Autodesk Fusion 360 part; units mm, degrees
note: some values were not read from the file. Chosen so that the rebuilt part matches the saved one: which bodies a step acts on.
(part 2 of 3)
  line L234 (-30.457, -45.4136) -> (-27.043, -43.5255) construction
  line L235 (-27.043, -43.5255) -> (-26.2697, -43.2195) construction
  spline S75 degree 3 poles (-26.2697, -43.2195) (-26.1288, -43.1638) (-26.0775, -43.1652) (-25.9254, -43.2288) knots 0 0 0 0 1 1 1 1
  line L236 (-26.2697, -43.2195) -> (-26.1288, -43.1638) construction
  line L237 (-26.1288, -43.1638) -> (-26.0775, -43.1652) construction
  line L238 (-26.0775, -43.1652) -> (-25.9254, -43.2288) construction
  spline S76 degree 3 poles (-25.9915, -44.0067) (-25.7575, -44.1128) (-24.8189, -44.5936) (-24.3388, -44.8532) knots 0 0 0 0 1 1 1 1
  line L239 (-25.9915, -44.0067) -> (-25.7575, -44.1128) construction
  line L240 (-25.7575, -44.1128) -> (-24.8189, -44.5936) construction
  line L241 (-24.8189, -44.5936) -> (-24.3388, -44.8532) construction
  spline S77 degree 3 poles (-24.3388, -44.8532) (-22.7885, -45.6916) (-21.6552, -46.3596) (-21.7503, -46.379) knots 0 0 0 0 1 1 1 1
  line L242 (-24.3388, -44.8532) -> (-22.7885, -45.6916) construction
  line L243 (-22.7885, -45.6916) -> (-21.6552, -46.3596) construction
  line L244 (-21.6552, -46.3596) -> (-21.7503, -46.379) construction
  spline S78 degree 3 poles (-21.7503, -46.379) (-21.829, -46.395) (-22.3918, -46.1318) (-24.2975, -45.188) knots 0 0 0 0 1 1 1 1
  line L245 (-21.7503, -46.379) -> (-21.829, -46.395) construction
  line L246 (-21.829, -46.395) -> (-22.3918, -46.1318) construction
  line L247 (-22.3918, -46.1318) -> (-24.2975, -45.188) construction
  spline S79 degree 3 poles (-24.2975, -45.188) (-25.1974, -44.7423) (-25.942, -44.3774) (-25.9521, -44.3772) knots 0 0 0 0 1 1 1 1
  line L248 (-24.2975, -45.188) -> (-25.1974, -44.7423) construction
  line L249 (-25.1974, -44.7423) -> (-25.942, -44.3774) construction
  line L250 (-25.942, -44.3774) -> (-25.9521, -44.3772) construction
  spline S80 degree 3 poles (-25.9521, -44.3772) (-25.9622, -44.3769) (-26.5014, -44.6487) (-27.1503, -44.981) knots 0 0 0 0 1 1 1 1
  line L251 (-25.9521, -44.3772) -> (-25.9622, -44.3769) construction
  line L252 (-25.9622, -44.3769) -> (-26.5014, -44.6487) construction
  line L253 (-26.5014, -44.6487) -> (-27.1503, -44.981) construction
  spline S81 degree 3 poles (-27.1503, -44.981) (-28.8926, -45.8734) (-29.5894, -46.2424) (-30.0354, -46.5089) knots 0 0 0 0 1 1 1 1
  line L254 (-27.1503, -44.981) -> (-28.8926, -45.8734) construction
  line L255 (-28.8926, -45.8734) -> (-29.5894, -46.2424) construction
  line L256 (-29.5894, -46.2424) -> (-30.0354, -46.5089) construction
  spline S82 degree 3 poles (-30.0354, -46.5089) (-30.1643, -46.586) (-30.3231, -46.667) (-30.3881, -46.689) knots 0 0 0 0 1 1 1 1
  line L257 (-30.0354, -46.5089) -> (-30.1643, -46.586) construction
  line L258 (-30.1643, -46.586) -> (-30.3231, -46.667) construction
  line L259 (-30.3231, -46.667) -> (-30.3881, -46.689) construction
  spline S83 degree 3 poles (-30.3881, -46.689) (-30.6444, -46.7757) (-30.8249, -46.7116) (-30.7157, -46.5728) knots 0 0 0 0 1 1 1 1
  line L260 (-30.3881, -46.689) -> (-30.6444, -46.7757) construction
  line L261 (-30.6444, -46.7757) -> (-30.8249, -46.7116) construction
  line L262 (-30.8249, -46.7116) -> (-30.7157, -46.5728) construction
  spline S84 degree 3 poles (-30.7157, -46.5728) (-30.5978, -46.4228) (-28.7477, -45.3044) (-27.2723, -44.491) knots 0 0 0 0 1 1 1 1
  line L263 (-30.7157, -46.5728) -> (-30.5978, -46.4228) construction
  line L264 (-30.5978, -46.4228) -> (-28.7477, -45.3044) construction
  line L265 (-28.7477, -45.3044) -> (-27.2723, -44.491) construction
  spline S85 degree 3 poles (-27.2723, -44.491) (-26.8574, -44.2623) (-26.2555, -43.9583) (-26.1898, -43.9443) knots 0 0 0 0 1 1 1 1
  line L266 (-27.2723, -44.491) -> (-26.8574, -44.2623) construction
  line L267 (-26.8574, -44.2623) -> (-26.2555, -43.9583) construction
  line L268 (-26.2555, -43.9583) -> (-26.1898, -43.9443) construction
  spline S86 degree 3 poles (-26.1898, -43.9443) (-26.1622, -43.9384) (-26.0966, -43.959) (-25.9915, -44.0067) knots 0 0 0 0 1 1 1 1
  line L269 (-26.1898, -43.9443) -> (-26.1622, -43.9384) construction
  line L270 (-26.1622, -43.9384) -> (-26.0966, -43.959) construction
  line L271 (-26.0966, -43.959) -> (-25.9915, -44.0067) construction
  spline S87 degree 3 poles (-26.0659, -44.7937) (-25.8421, -44.8752) (-25.0562, -45.2692) (-24.3884, -45.6347) knots 0 0 0 0 1 1 1 1
  line L272 (-26.0659, -44.7937) -> (-25.8421, -44.8752) construction
  line L273 (-25.8421, -44.8752) -> (-25.0562, -45.2692) construction
  line L274 (-25.0562, -45.2692) -> (-24.3884, -45.6347) construction
  spline S88 degree 3 poles (-24.3884, -45.6347) (-23.4262, -46.1613) (-22.272, -46.841) (-22.1077, -46.9777) knots 0 0 0 0 1 1 1 1
  line L275 (-24.3884, -45.6347) -> (-23.4262, -46.1613) construction
  line L276 (-23.4262, -46.1613) -> (-22.272, -46.841) construction
  line L277 (-22.272, -46.841) -> (-22.1077, -46.9777) construction
  line L278 (-22.1077, -46.9777) -> (-22.0664, -47.0121)
  line L279 (-22.0664, -47.0121) -> (-22.1077, -47.0012)
  spline S89 degree 3 poles (-22.1077, -47.0012) (-22.1774, -46.9831) (-22.6584, -46.7746) (-23.0415, -46.5965) knots 0 0 0 0 1 1 1 1
  line L280 (-22.1077, -47.0012) -> (-22.1774, -46.9831) construction
  line L281 (-22.1774, -46.9831) -> (-22.6584, -46.7746) construction
  line L282 (-22.6584, -46.7746) -> (-23.0415, -46.5965) construction
  spline S90 degree 3 poles (-23.0415, -46.5965) (-23.2415, -46.5036) (-23.9837, -46.1421) (-24.691, -45.7932) knots 0 0 0 0 1 1 1 1
  line L283 (-23.0415, -46.5965) -> (-23.2415, -46.5036) construction
  line L284 (-23.2415, -46.5036) -> (-23.9837, -46.1421) construction
  line L285 (-23.9837, -46.1421) -> (-24.691, -45.7932) construction
  spline S91 degree 3 poles (-24.691, -45.7932) (-25.3982, -45.4444) (-25.9848, -45.159) (-25.9944, -45.159) knots 0 0 0 0 1 1 1 1
  line L286 (-24.691, -45.7932) -> (-25.3982, -45.4444) construction
  line L287 (-25.3982, -45.4444) -> (-25.9848, -45.159) construction
  line L288 (-25.9848, -45.159) -> (-25.9944, -45.159) construction
  spline S92 degree 3 poles (-25.9944, -45.159) (-26.0041, -45.159) (-26.5075, -45.4221) (-27.1131, -45.7436) knots 0 0 0 0 1 1 1 1
  line L289 (-25.9944, -45.159) -> (-26.0041, -45.159) construction
  line L290 (-26.0041, -45.159) -> (-26.5075, -45.4221) construction
  line L291 (-26.5075, -45.4221) -> (-27.1131, -45.7436) construction
  spline S93 degree 3 poles (-27.1131, -45.7436) (-29.2269, -46.8659) (-30.1751, -47.357) (-30.2282, -47.357) knots 0 0 0 0 1 1 1 1
  line L292 (-27.1131, -45.7436) -> (-29.2269, -46.8659) construction
  line L293 (-29.2269, -46.8659) -> (-30.1751, -47.357) construction
  line L294 (-30.1751, -47.357) -> (-30.2282, -47.357) construction
  spline S94 degree 3 poles (-30.2282, -47.357) (-30.2637, -47.357) (-30.2915, -47.2851) (-30.2851, -47.2098) knots 0 0 0 0 1 1 1 1
  line L295 (-30.2282, -47.357) -> (-30.2637, -47.357) construction
  line L296 (-30.2637, -47.357) -> (-30.2915, -47.2851) construction
  line L297 (-30.2915, -47.2851) -> (-30.2851, -47.2098) construction
  spline S95 degree 3 poles (-30.2851, -47.2098) (-30.281, -47.1611) (-30.2639, -47.1384) (-30.181, -47.0712) knots 0 0 0 0 1 1 1 1
  line L298 (-30.2851, -47.2098) -> (-30.281, -47.1611) construction
  line L299 (-30.281, -47.1611) -> (-30.2639, -47.1384) construction
  line L300 (-30.2639, -47.1384) -> (-30.181, -47.0712) construction
  spline S96 degree 3 poles (-30.181, -47.0712) (-29.6415, -46.6342) (-26.8805, -45.0293) (-26.2762, -44.8014) knots 0 0 0 0 1 1 1 1
  line L301 (-30.181, -47.0712) -> (-29.6415, -46.6342) construction
  line L302 (-29.6415, -46.6342) -> (-26.8805, -45.0293) construction
  line L303 (-26.8805, -45.0293) -> (-26.2762, -44.8014) construction
  spline S97 degree 3 poles (-26.2762, -44.8014) (-26.154, -44.7553) (-26.1694, -44.7559) (-26.0659, -44.7937) knots 0 0 0 0 1 1 1 1
  line L304 (-26.2762, -44.8014) -> (-26.154, -44.7553) construction
  line L305 (-26.154, -44.7553) -> (-26.1694, -44.7559) construction
  line L306 (-26.1694, -44.7559) -> (-26.0659, -44.7937) construction
  spline S98 degree 3 poles (-25.8841, -45.7204) (-25.6348, -45.7864) (-25.4625, -45.8734) (-24.2727, -46.5342) knots 0 0 0 0 1 1 1 1
  line L307 (-25.8841, -45.7204) -> (-25.6348, -45.7864) construction
  line L308 (-25.6348, -45.7864) -> (-25.4625, -45.8734) construction
  line L309 (-25.4625, -45.8734) -> (-24.2727, -46.5342) construction
  spline S99 degree 3 poles (-24.2727, -46.5342) (-23.1246, -47.1718) (-22.3847, -47.6206) (-22.4583, -47.6347) knots 0 0 0 0 1 1 1 1
  line L310 (-24.2727, -46.5342) -> (-23.1246, -47.1718) construction
  line L311 (-23.1246, -47.1718) -> (-22.3847, -47.6206) construction
  line L312 (-22.3847, -47.6206) -> (-22.4583, -47.6347) construction
  spline S100 degree 3 poles (-22.4583, -47.6347) (-22.4937, -47.6415) (-22.7889, -47.5251) (-23.1407, -47.3656) knots 0 0 0 0 1 1 1 1
  line L313 (-22.4583, -47.6347) -> (-22.4937, -47.6415) construction
  line L314 (-22.4937, -47.6415) -> (-22.7889, -47.5251) construction
  line L315 (-22.7889, -47.5251) -> (-23.1407, -47.3656) construction
  spline S101 degree 3 poles (-23.1407, -47.3656) (-23.4951, -47.2048) (-24.3025, -46.8056) (-25.2404, -46.3275) knots 0 0 0 0 1 1 1 1
  line L316 (-23.1407, -47.3656) -> (-23.4951, -47.2048) construction
  line L317 (-23.4951, -47.2048) -> (-24.3025, -46.8056) construction
  line L318 (-24.3025, -46.8056) -> (-25.2404, -46.3275) construction
  line L319 (-25.2404, -46.3275) -> (-25.9684, -45.9564)
  line L320 (-25.9684, -45.9564) -> (-26.9591, -46.4853)
  spline S102 degree 3 poles (-26.9591, -46.4853) (-28.0366, -47.0606) (-29.1621, -47.6344) (-29.4601, -47.7604) knots 0 0 0 0 1 1 1 1
  line L321 (-26.9591, -46.4853) -> (-28.0366, -47.0606) construction
  line L322 (-28.0366, -47.0606) -> (-29.1621, -47.6344) construction
  line L323 (-29.1621, -47.6344) -> (-29.4601, -47.7604) construction
  spline S103 degree 3 poles (-29.4601, -47.7604) (-29.6667, -47.8478) (-29.7412, -47.8533) (-29.7967, -47.7854) knots 0 0 0 0 1 1 1 1
  line L324 (-29.4601, -47.7604) -> (-29.6667, -47.8478) construction
  line L325 (-29.6667, -47.8478) -> (-29.7412, -47.8533) construction
  line L326 (-29.7412, -47.8533) -> (-29.7967, -47.7854) construction
  spline S104 degree 3 poles (-29.7967, -47.7854) (-29.8338, -47.74) (-29.8332, -47.7011) (-29.7942, -47.625) knots 0 0 0 0 1 1 1 1
  line L327 (-29.7967, -47.7854) -> (-29.8338, -47.74) construction
  line L328 (-29.8338, -47.74) -> (-29.8332, -47.7011) construction
  line L329 (-29.8332, -47.7011) -> (-29.7942, -47.625) construction
  spline S105 degree 3 poles (-29.7942, -47.625) (-29.7453, -47.5297) (-29.7064, -47.5026) (-29.3794, -47.3363) knots 0 0 0 0 1 1 1 1
  line L330 (-29.7942, -47.625) -> (-29.7453, -47.5297) construction
  line L331 (-29.7453, -47.5297) -> (-29.7064, -47.5026) construction
  line L332 (-29.7064, -47.5026) -> (-29.3794, -47.3363) construction
  spline S106 degree 3 poles (-29.3794, -47.3363) (-28.995, -47.1408) (-28.5135, -46.8671) (-27.7433, -46.4059) knots 0 0 0 0 1 1 1 1
  line L333 (-29.3794, -47.3363) -> (-28.995, -47.1408) construction
  line L334 (-28.995, -47.1408) -> (-28.5135, -46.8671) construction
  line L335 (-28.5135, -46.8671) -> (-27.7433, -46.4059) construction
  spline S107 degree 3 poles (-27.7433, -46.4059) (-27.0552, -45.994) (-26.6414, -45.7766) (-26.4448, -45.7237) knots 0 0 0 0 1 1 1 1
  line L336 (-27.7433, -46.4059) -> (-27.0552, -45.994) construction
  line L337 (-27.0552, -45.994) -> (-26.6414, -45.7766) construction
  line L338 (-26.6414, -45.7766) -> (-26.4448, -45.7237) construction
  spline S108 degree 3 poles (-26.4448, -45.7237) (-26.2751, -45.6781) (-26.0486, -45.6767) (-25.8841, -45.7204) knots 0 0 0 0 1 1 1 1
  line L339 (-26.4448, -45.7237) -> (-26.2751, -45.6781) construction
  line L340 (-26.2751, -45.6781) -> (-26.0486, -45.6767) construction
  line L341 (-26.0486, -45.6767) -> (-25.8841, -45.7204) construction
  spline S109 degree 3 poles (-25.8722, -46.4976) (-25.704, -46.5545) (-25.5311, -46.6392) (-25.2843, -46.7853) knots 0 0 0 0 1 1 1 1
  line L342 (-25.8722, -46.4976) -> (-25.704, -46.5545) construction
  line L343 (-25.704, -46.5545) -> (-25.5311, -46.6392) construction
  line L344 (-25.5311, -46.6392) -> (-25.2843, -46.7853) construction
  spline S110 degree 3 poles (-25.2843, -46.7853) (-25.0154, -46.9446) (-24.4604, -47.2593) (-24, -47.5135) knots 0 0 0 0 1 1 1 1
  line L345 (-25.2843, -46.7853) -> (-25.0154, -46.9446) construction
  line L346 (-25.0154, -46.9446) -> (-24.4604, -47.2593) construction
  line L347 (-24.4604, -47.2593) -> (-24, -47.5135) construction
  spline S111 degree 3 poles (-24, -47.5135) (-23.313, -47.8929) (-22.9534, -48.1126) (-22.8762, -48.2001) knots 0 0 0 0 1 1 1 1
  line L348 (-24, -47.5135) -> (-23.313, -47.8929) construction
  line L349 (-23.313, -47.8929) -> (-22.9534, -48.1126) construction
  line L350 (-22.9534, -48.1126) -> (-22.8762, -48.2001) construction
  line L351 (-22.8762, -48.2001) -> (-22.8432, -48.2376)
  line L352 (-22.8432, -48.2376) -> (-22.9087, -48.2256)
  spline S112 degree 3 poles (-22.9087, -48.2256) (-23.1186, -48.1871) (-23.6529, -47.9448) (-24.9223, -47.3123) knots 0 0 0 0 1 1 1 1
  line L353 (-22.9087, -48.2256) -> (-23.1186, -48.1871) construction
  line L354 (-23.1186, -48.1871) -> (-23.6529, -47.9448) construction
  line L355 (-23.6529, -47.9448) -> (-24.9223, -47.3123) construction
  spline S113 degree 3 poles (-24.9223, -47.3123) (-25.475, -47.037) (-25.9351, -46.8117) (-25.9447, -46.8117) knots 0 0 0 0 1 1 1 1
  line L356 (-24.9223, -47.3123) -> (-25.475, -47.037) construction
  line L357 (-25.475, -47.037) -> (-25.9351, -46.8117) construction
  line L358 (-25.9351, -46.8117) -> (-25.9447, -46.8117) construction
  spline S114 degree 3 poles (-25.9447, -46.8117) (-25.9544, -46.8117) (-26.2794, -46.9746) (-26.6669, -47.1737) knots 0 0 0 0 1 1 1 1
  line L359 (-25.9447, -46.8117) -> (-25.9544, -46.8117) construction
  line L360 (-25.9544, -46.8117) -> (-26.2794, -46.9746) construction
  line L361 (-26.2794, -46.9746) -> (-26.6669, -47.1737) construction
  spline S115 degree 3 poles (-26.6669, -47.1737) (-28.0497, -47.8842) (-28.5938, -48.1478) (-29.0112, -48.3091) knots 0 0 0 0 1 1 1 1
  line L362 (-26.6669, -47.1737) -> (-28.0497, -47.8842) construction
  line L363 (-28.0497, -47.8842) -> (-28.5938, -48.1478) construction
  line L364 (-28.5938, -48.1478) -> (-29.0112, -48.3091) construction
  spline S116 degree 3 poles (-29.0112, -48.3091) (-29.1142, -48.3489) (-29.2276, -48.3861) (-29.2633, -48.3918) knots 0 0 0 0 1 1 1 1
  line L365 (-29.0112, -48.3091) -> (-29.1142, -48.3489) construction
  line L366 (-29.1142, -48.3489) -> (-29.2276, -48.3861) construction
  line L367 (-29.2276, -48.3861) -> (-29.2633, -48.3918) construction
  spline S117 degree 3 poles (-29.2633, -48.3918) (-29.3229, -48.4013) (-29.3291, -48.3987) (-29.3388, -48.3601) knots 0 0 0 0 1 1 1 1
  line L368 (-29.2633, -48.3918) -> (-29.3229, -48.4013) construction
  line L369 (-29.3229, -48.4013) -> (-29.3291, -48.3987) construction
  line L370 (-29.3291, -48.3987) -> (-29.3388, -48.3601) construction
  spline S118 degree 3 poles (-29.3388, -48.3601) (-29.3638, -48.2604) (-29.29, -48.1741) (-29.033, -48.0024) knots 0 0 0 0 1 1 1 1
  line L371 (-29.3388, -48.3601) -> (-29.3638, -48.2604) construction
  line L372 (-29.3638, -48.2604) -> (-29.29, -48.1741) construction
  line L373 (-29.29, -48.1741) -> (-29.033, -48.0024) construction
  spline S119 degree 3 poles (-29.033, -48.0024) (-28.4019, -47.5806) (-26.7702, -46.6937) (-26.2531, -46.4912) knots 0 0 0 0 1 1 1 1
  line L374 (-29.033, -48.0024) -> (-28.4019, -47.5806) construction
  line L375 (-28.4019, -47.5806) -> (-26.7702, -46.6937) construction
  line L376 (-26.7702, -46.6937) -> (-26.2531, -46.4912) construction
  spline S120 degree 3 poles (-26.2531, -46.4912) (-26.1127, -46.4363) (-26.05, -46.4373) (-25.8722, -46.4976) knots 0 0 0 0 1 1 1 1
  line L377 (-26.2531, -46.4912) -> (-26.1127, -46.4363) construction
  line L378 (-26.1127, -46.4363) -> (-26.05, -46.4373) construction
  line L379 (-26.05, -46.4373) -> (-25.8722, -46.4976) construction
  spline S121 degree 3 poles (-26.0328, -47.2597) (-25.9016, -47.3132) (-25.2551, -47.6361) (-24.8759, -47.8375) knots 0 0 0 0 1 1 1 1
  line L380 (-26.0328, -47.2597) -> (-25.9016, -47.3132) construction
  line L381 (-25.9016, -47.3132) -> (-25.2551, -47.6361) construction
  line L382 (-25.2551, -47.6361) -> (-24.8759, -47.8375) construction
  spline S122 degree 3 poles (-24.8759, -47.8375) (-24.0296, -48.287) (-23.2843, -48.7426) (-23.3689, -48.7589) knots 0 0 0 0 1 1 1 1
  line L383 (-24.8759, -47.8375) -> (-24.0296, -48.287) construction
  line L384 (-24.0296, -48.287) -> (-23.2843, -48.7426) construction
  line L385 (-23.2843, -48.7426) -> (-23.3689, -48.7589) construction
  spline S123 degree 3 poles (-23.3689, -48.7589) (-23.4678, -48.7779) (-24.1054, -48.5) (-25.271, -47.9296) knots 0 0 0 0 1 1 1 1
  line L386 (-23.3689, -48.7589) -> (-23.4678, -48.7779) construction
  line L387 (-23.4678, -48.7779) -> (-24.1054, -48.5) construction
  line L388 (-24.1054, -48.5) -> (-25.271, -47.9296) construction
  spline S124 degree 3 poles (-25.271, -47.9296) (-25.7194, -47.7101) (-25.9049, -47.627) (-25.9238, -47.6371) knots 0 0 0 0 1 1 1 1
  line L389 (-25.271, -47.9296) -> (-25.7194, -47.7101) construction
  line L390 (-25.7194, -47.7101) -> (-25.9049, -47.627) construction
  line L391 (-25.9049, -47.627) -> (-25.9238, -47.6371) construction
  spline S125 degree 3 poles (-25.9238, -47.6371) (-25.9986, -47.6768) (-27.5715, -48.4353) (-27.7846, -48.5344) knots 0 0 0 0 1 1 1 1
  line L392 (-25.9238, -47.6371) -> (-25.9986, -47.6768) construction
  line L393 (-25.9986, -47.6768) -> (-27.5715, -48.4353) construction
  line L394 (-27.5715, -48.4353) -> (-27.7846, -48.5344) construction
  spline S126 degree 3 poles (-27.7846, -48.5344) (-28.514, -48.8736) (-28.7769, -48.9621) (-28.8571, -48.8955) knots 0 0 0 0 1 1 1 1
  line L395 (-27.7846, -48.5344) -> (-28.514, -48.8736) construction
  line L396 (-28.514, -48.8736) -> (-28.7769, -48.9621) construction
  line L397 (-28.7769, -48.9621) -> (-28.8571, -48.8955) construction
  spline S127 degree 3 poles (-28.8571, -48.8955) (-28.9273, -48.8372) (-28.8768, -48.7847) (-28.5319, -48.5575) knots 0 0 0 0 1 1 1 1
  line L398 (-28.8571, -48.8955) -> (-28.9273, -48.8372) construction
  line L399 (-28.9273, -48.8372) -> (-28.8768, -48.7847) construction
  line L400 (-28.8768, -48.7847) -> (-28.5319, -48.5575) construction
  spline S128 degree 3 poles (-28.5319, -48.5575) (-27.7923, -48.0703) (-26.3775, -47.2824) (-26.1567, -47.2348) knots 0 0 0 0 1 1 1 1
  line L401 (-28.5319, -48.5575) -> (-27.7923, -48.0703) construction
  line L402 (-27.7923, -48.0703) -> (-26.3775, -47.2824) construction
  line L403 (-26.3775, -47.2824) -> (-26.1567, -47.2348) construction
  spline S129 degree 3 poles (-26.1567, -47.2348) (-26.1335, -47.2299) (-26.0794, -47.2407) (-26.0328, -47.2597) knots 0 0 0 0 1 1 1 1
  line L404 (-26.1567, -47.2348) -> (-26.1335, -47.2299) construction
  line L405 (-26.1335, -47.2299) -> (-26.0794, -47.2407) construction
  line L406 (-26.0794, -47.2407) -> (-26.0328, -47.2597) construction
  spline S130 degree 3 poles (-25.9006, -48.1072) (-25.2283, -48.4297) (-23.942, -49.1704) (-23.8197, -49.3056) knots 0 0 0 0 1 1 1 1
  line L407 (-25.9006, -48.1072) -> (-25.2283, -48.4297) construction
  line L408 (-25.2283, -48.4297) -> (-23.942, -49.1704) construction
  line L409 (-23.942, -49.1704) -> (-23.8197, -49.3056) construction
  spline S131 degree 3 poles (-23.8197, -49.3056) (-23.7888, -49.3397) (-23.7889, -49.3402) (-23.8227, -49.3402) knots 0 0 0 0 1 1 1 1
  line L410 (-23.8197, -49.3056) -> (-23.7888, -49.3397) construction
  line L411 (-23.7888, -49.3397) -> (-23.7889, -49.3402) construction
  line L412 (-23.7889, -49.3402) -> (-23.8227, -49.3402) construction
  spline S132 degree 3 poles (-23.8227, -49.3402) (-23.9179, -49.3402) (-24.4007, -49.144) (-25.2495, -48.7602) knots 0 0 0 0 1 1 1 1
  line L413 (-23.8227, -49.3402) -> (-23.9179, -49.3402) construction
  line L414 (-23.9179, -49.3402) -> (-24.4007, -49.144) construction
  line L415 (-24.4007, -49.144) -> (-25.2495, -48.7602) construction
  spline S133 degree 3 poles (-25.2495, -48.7602) (-25.6094, -48.5975) (-25.913, -48.4643) (-25.924, -48.4643) knots 0 0 0 0 1 1 1 1
  line L416 (-25.2495, -48.7602) -> (-25.6094, -48.5975) construction
  line L417 (-25.6094, -48.5975) -> (-25.913, -48.4643) construction
  line L418 (-25.913, -48.4643) -> (-25.924, -48.4643) construction
  spline S134 degree 3 poles (-25.924, -48.4643) (-25.935, -48.4643) (-26.2244, -48.5991) (-26.5669, -48.7639) knots 0 0 0 0 1 1 1 1
  line L419 (-25.924, -48.4643) -> (-25.935, -48.4643) construction
  line L420 (-25.935, -48.4643) -> (-26.2244, -48.5991) construction
  line L421 (-26.2244, -48.5991) -> (-26.5669, -48.7639) construction
  spline S135 degree 3 poles (-26.5669, -48.7639) (-27.3036, -49.1182) (-27.5407, -49.2246) (-27.849, -49.3392) knots 0 0 0 0 1 1 1 1
  line L422 (-26.5669, -48.7639) -> (-27.3036, -49.1182) construction
  line L423 (-27.3036, -49.1182) -> (-27.5407, -49.2246) construction
  line L424 (-27.5407, -49.2246) -> (-27.849, -49.3392) construction
  spline S136 degree 3 poles (-27.849, -49.3392) (-28.0734, -49.4226) (-28.3094, -49.4887) (-28.3838, -49.4889) knots 0 0 0 0 1 1 1 1
  line L425 (-27.849, -49.3392) -> (-28.0734, -49.4226) construction
  line L426 (-28.0734, -49.4226) -> (-28.3094, -49.4887) construction
  line L427 (-28.3094, -49.4887) -> (-28.3838, -49.4889) construction
  spline S137 degree 3 poles (-28.3838, -49.4889) (-28.5219, -49.4894) (-28.2585, -49.2609) (-27.669, -48.8691) knots 0 0 0 0 1 1 1 1
  line L428 (-28.3838, -49.4889) -> (-28.5219, -49.4894) construction
  line L429 (-28.5219, -49.4894) -> (-28.2585, -49.2609) construction
  line L430 (-28.2585, -49.2609) -> (-27.669, -48.8691) construction
  spline S138 degree 3 poles (-27.669, -48.8691) (-26.9446, -48.3877) (-26.2659, -48.0154) (-26.1193, -48.0191) knots 0 0 0 0 1 1 1 1
  line L431 (-27.669, -48.8691) -> (-26.9446, -48.3877) construction
  line L432 (-26.9446, -48.3877) -> (-26.2659, -48.0154) construction
  line L433 (-26.2659, -48.0154) -> (-26.1193, -48.0191) construction
  spline S139 degree 3 poles (-26.1193, -48.0191) (-26.099, -48.0195) (-26.0006, -48.0592) (-25.9006, -48.1072) knots 0 0 0 0 1 1 1 1
  line L434 (-26.1193, -48.0191) -> (-26.099, -48.0195) construction
  line L435 (-26.099, -48.0195) -> (-26.0006, -48.0592) construction
  line L436 (-26.0006, -48.0592) -> (-25.9006, -48.1072) construction
  spline S140 degree 3 poles (-25.9254, -48.9692) (-25.8145, -48.9977) (-24.4971, -49.6532) (-24.3171, -49.7694) knots 0 0 0 0 1 1 1 1
  line L437 (-25.9254, -48.9692) -> (-25.8145, -48.9977) construction
  line L438 (-25.8145, -48.9977) -> (-24.4971, -49.6532) construction
  line L439 (-24.4971, -49.6532) -> (-24.3171, -49.7694) construction
  spline S141 degree 3 poles (-24.3171, -49.7694) (-24.202, -49.8437) (-24.1885, -49.8578) (-24.1931, -49.8982) knots 0 0 0 0 1 1 1 1
  line L440 (-24.3171, -49.7694) -> (-24.202, -49.8437) construction
  line L441 (-24.202, -49.8437) -> (-24.1885, -49.8578) construction
  line L442 (-24.1885, -49.8578) -> (-24.1931, -49.8982) construction
  spline S142 degree 3 poles (-24.1931, -49.8982) (-24.2002, -49.959) (-24.2445, -49.9635) (-24.3936, -49.9184) knots 0 0 0 0 1 1 1 1
  line L443 (-24.1931, -49.8982) -> (-24.2002, -49.959) construction
  line L444 (-24.2002, -49.959) -> (-24.2445, -49.9635) construction
  line L445 (-24.2445, -49.9635) -> (-24.3936, -49.9184) construction
  spline S143 degree 3 poles (-24.3936, -49.9184) (-24.5983, -49.8565) (-24.875, -49.7409) (-25.4105, -49.4935) knots 0 0 0 0 1 1 1 1
  line L446 (-24.3936, -49.9184) -> (-24.5983, -49.8565) construction
  line L447 (-24.5983, -49.8565) -> (-24.875, -49.7409) construction
  line L448 (-24.875, -49.7409) -> (-25.4105, -49.4935) construction
  line L449 (-25.4105, -49.4935) -> (-25.9286, -49.2542)
  line L450 (-25.9286, -49.2542) -> (-26.5095, -49.5354)
  spline S144 degree 3 poles (-26.5095, -49.5354) (-27.3555, -49.9449) (-27.6003, -50.0371) (-27.8507, -50.0406) knots 0 0 0 0 1 1 1 1
  line L451 (-26.5095, -49.5354) -> (-27.3555, -49.9449) construction
  line L452 (-27.3555, -49.9449) -> (-27.6003, -50.0371) construction
  line L453 (-27.6003, -50.0371) -> (-27.8507, -50.0406) construction
  spline S145 degree 3 poles (-27.8507, -50.0406) (-27.9926, -50.0425) (-27.9997, -50.0409) (-28.0047, -50.0059) knots 0 0 0 0 1 1 1 1
  line L454 (-27.8507, -50.0406) -> (-27.9926, -50.0425) construction
  line L455 (-27.9926, -50.0425) -> (-27.9997, -50.0409) construction
  line L456 (-27.9997, -50.0409) -> (-28.0047, -50.0059) construction
  spline S146 degree 3 poles (-28.0047, -50.0059) (-28.012, -49.9538) (-27.8877, -49.8263) (-27.7128, -49.7065) knots 0 0 0 0 1 1 1 1
  line L457 (-28.0047, -50.0059) -> (-28.012, -49.9538) construction
  line L458 (-28.012, -49.9538) -> (-27.8877, -49.8263) construction
  line L459 (-27.8877, -49.8263) -> (-27.7128, -49.7065) construction
  spline S147 degree 3 poles (-27.7128, -49.7065) (-27.5513, -49.596) (-26.8845, -49.2091) (-26.6652, -49.0988) knots 0 0 0 0 1 1 1 1
  line L460 (-27.7128, -49.7065) -> (-27.5513, -49.596) construction
  line L461 (-27.5513, -49.596) -> (-26.8845, -49.2091) construction
  line L462 (-26.8845, -49.2091) -> (-26.6652, -49.0988) construction
  spline S148 degree 3 poles (-26.6652, -49.0988) (-26.3641, -48.9473) (-26.1537, -48.9104) (-25.9254, -48.9692) knots 0 0 0 0 1 1 1 1
  line L463 (-26.6652, -49.0988) -> (-26.3641, -48.9473) construction
  line L464 (-26.3641, -48.9473) -> (-26.1537, -48.9104) construction
  line L465 (-26.1537, -48.9104) -> (-25.9254, -48.9692) construction
  spline S149 degree 3 poles (-25.8427, -49.7941) (-25.6795, -49.8407) (-25.3299, -50.0067) (-25.0638, -50.164) knots 0 0 0 0 1 1 1 1
  line L466 (-25.8427, -49.7941) -> (-25.6795, -49.8407) construction
  line L467 (-25.6795, -49.8407) -> (-25.3299, -50.0067) construction
  line L468 (-25.3299, -50.0067) -> (-25.0638, -50.164) construction
  spline S150 degree 3 poles (-25.0638, -50.164) (-24.796, -50.3224) (-24.6972, -50.4481) (-24.8306, -50.461) knots 0 0 0 0 1 1 1 1
  line L469 (-25.0638, -50.164) -> (-24.796, -50.3224) construction
  line L470 (-24.796, -50.3224) -> (-24.6972, -50.4481) construction
  line L471 (-24.6972, -50.4481) -> (-24.8306, -50.461) construction
  spline S151 degree 3 poles (-24.8306, -50.461) (-24.9117, -50.4688) (-25.1331, -50.4077) (-25.3984, -50.3043) knots 0 0 0 0 1 1 1 1
  line L472 (-24.8306, -50.461) -> (-24.9117, -50.4688) construction
  line L473 (-24.9117, -50.4688) -> (-25.1331, -50.4077) construction
  line L474 (-25.1331, -50.4077) -> (-25.3984, -50.3043) construction
  spline S152 degree 3 poles (-25.3984, -50.3043) (-25.699, -50.1871) (-25.7745, -50.167) (-25.9147, -50.1668) knots 0 0 0 0 1 1 1 1
  line L475 (-25.3984, -50.3043) -> (-25.699, -50.1871) construction
  line L476 (-25.699, -50.1871) -> (-25.7745, -50.167) construction
  line L477 (-25.7745, -50.167) -> (-25.9147, -50.1668) construction
  spline S153 degree 3 poles (-25.9147, -50.1668) (-26.0765, -50.1665) (-26.1933, -50.2019) (-26.5139, -50.3483) knots 0 0 0 0 1 1 1 1
  line L478 (-25.9147, -50.1668) -> (-26.0765, -50.1665) construction
  line L479 (-26.0765, -50.1665) -> (-26.1933, -50.2019) construction
  line L480 (-26.1933, -50.2019) -> (-26.5139, -50.3483) construction
  spline S154 degree 3 poles (-26.5139, -50.3483) (-26.9633, -50.5536) (-27.2052, -50.6374) (-27.4045, -50.6567) knots 0 0 0 0 1 1 1 1
  line L481 (-26.5139, -50.3483) -> (-26.9633, -50.5536) construction
  line L482 (-26.9633, -50.5536) -> (-27.2052, -50.6374) construction
  line L483 (-27.2052, -50.6374) -> (-27.4045, -50.6567) construction
  spline S155 degree 3 poles (-27.4045, -50.6567) (-27.4871, -50.6646) (-27.5102, -50.6609) (-27.5429, -50.6344) knots 0 0 0 0 1 1 1 1
  line L484 (-27.4045, -50.6567) -> (-27.4871, -50.6646) construction
  line L485 (-27.4871, -50.6646) -> (-27.5102, -50.6609) construction
  line L486 (-27.5102, -50.6609) -> (-27.5429, -50.6344) construction
  spline S156 degree 3 poles (-27.5429, -50.6344) (-27.5806, -50.6038) (-27.5811, -50.6005) (-27.556, -50.552) knots 0 0 0 0 1 1 1 1
  line L487 (-27.5429, -50.6344) -> (-27.5806, -50.6038) construction
  line L488 (-27.5806, -50.6038) -> (-27.5811, -50.6005) construction
  line L489 (-27.5811, -50.6005) -> (-27.556, -50.552) construction
  spline S157 degree 3 poles (-27.556, -50.552) (-27.5229, -50.4881) (-27.3926, -50.3704) (-27.2502, -50.276) knots 0 0 0 0 1 1 1 1
  line L490 (-27.556, -50.552) -> (-27.5229, -50.4881) construction
  line L491 (-27.5229, -50.4881) -> (-27.3926, -50.3704) construction
  line L492 (-27.3926, -50.3704) -> (-27.2502, -50.276) construction
  spline S158 degree 3 poles (-27.2502, -50.276) (-26.9831, -50.0988) (-26.4712, -49.8463) (-26.2771, -49.796) knots 0 0 0 0 1 1 1 1
  line L493 (-27.2502, -50.276) -> (-26.9831, -50.0988) construction
  line L494 (-26.9831, -50.0988) -> (-26.4712, -49.8463) construction
  line L495 (-26.4712, -49.8463) -> (-26.2771, -49.796) construction
  spline S159 degree 3 poles (-26.2771, -49.796) (-26.1585, -49.7652) (-25.9473, -49.7643) (-25.8427, -49.7941) knots 0 0 0 0 1 1 1 1
  line L496 (-26.2771, -49.796) -> (-26.1585, -49.7652) construction
  line L497 (-26.1585, -49.7652) -> (-25.9473, -49.7643) construction
  line L498 (-25.9473, -49.7643) -> (-25.8427, -49.7941) construction
  spline S160 degree 3 poles (-26.0163, -50.55) (-25.7916, -50.6279) (-25.2799, -50.9167) (-25.2232, -50.9977) knots 0 0 0 0 1 1 1 1
  line L499 (-26.0163, -50.55) -> (-25.7916, -50.6279) construction
  line L500 (-25.7916, -50.6279) -> (-25.2799, -50.9167) construction
  line L501 (-25.2799, -50.9167) -> (-25.2232, -50.9977) construction
  spline S161 degree 3 poles (-25.2232, -50.9977) (-25.143, -51.1121) (-25.2749, -51.1127) (-25.6038, -50.9992) knots 0 0 0 0 1 1 1 1
  line L502 (-25.2232, -50.9977) -> (-25.143, -51.1121) construction
  line L503 (-25.143, -51.1121) -> (-25.2749, -51.1127) construction
  line L504 (-25.2749, -51.1127) -> (-25.6038, -50.9992) construction
  spline S162 degree 3 poles (-25.6038, -50.9992) (-25.713, -50.9615) (-25.7633, -50.9538) (-25.9006, -50.9538) knots 0 0 0 0 1 1 1 1
  line L505 (-25.6038, -50.9992) -> (-25.713, -50.9615) construction
  line L506 (-25.713, -50.9615) -> (-25.7633, -50.9538) construction
  line L507 (-25.7633, -50.9538) -> (-25.9006, -50.9538) construction
  spline S163 degree 3 poles (-25.9006, -50.9538) (-26.0871, -50.9538) (-26.2188, -50.9903) (-26.4505, -51.1065) knots 0 0 0 0 1 1 1 1
  line L508 (-25.9006, -50.9538) -> (-26.0871, -50.9538) construction
  line L509 (-26.0871, -50.9538) -> (-26.2188, -50.9903) construction
  line L510 (-26.2188, -50.9903) -> (-26.4505, -51.1065) construction
  spline S164 degree 3 poles (-26.4505, -51.1065) (-26.7236, -51.2434) (-26.9716, -51.3032) (-27.0801, -51.2582) knots 0 0 0 0 1 1 1 1
  line L511 (-26.4505, -51.1065) -> (-26.7236, -51.2434) construction
  line L512 (-26.7236, -51.2434) -> (-26.9716, -51.3032) construction
  line L513 (-26.9716, -51.3032) -> (-27.0801, -51.2582) construction
  spline S165 degree 3 poles (-27.0801, -51.2582) (-27.1388, -51.2339) (-27.1754, -51.1592) (-27.151, -51.1135) knots 0 0 0 0 1 1 1 1
  line L514 (-27.0801, -51.2582) -> (-27.1388, -51.2339) construction
  line L515 (-27.1388, -51.2339) -> (-27.1754, -51.1592) construction
  line L516 (-27.1754, -51.1592) -> (-27.151, -51.1135) construction
  spline S166 degree 3 poles (-27.151, -51.1135) (-27.0975, -51.0135) (-26.8146, -50.8094) (-26.5369, -50.6703) knots 0 0 0 0 1 1 1 1
  line L517 (-27.151, -51.1135) -> (-27.0975, -51.0135) construction
  line L518 (-27.0975, -51.0135) -> (-26.8146, -50.8094) construction
  line L519 (-26.8146, -50.8094) -> (-26.5369, -50.6703) construction
  spline S167 degree 3 poles (-26.5369, -50.6703) (-26.2672, -50.5353) (-26.142, -50.5064) (-26.0163, -50.55) knots 0 0 0 0 1 1 1 1
  line L520 (-26.5369, -50.6703) -> (-26.2672, -50.5353) construction
  line L521 (-26.2672, -50.5353) -> (-26.142, -50.5064) construction
  line L522 (-26.142, -50.5064) -> (-26.0163, -50.55) construction
  spline S168 degree 3 poles (-25.8871, -51.3719) (-25.816, -51.3976) (-25.7354, -51.4399) (-25.7079, -51.466) knots 0 0 0 0 1 1 1 1
  line L523 (-25.8871, -51.3719) -> (-25.816, -51.3976) construction
  line L524 (-25.816, -51.3976) -> (-25.7354, -51.4399) construction
  line L525 (-25.7354, -51.4399) -> (-25.7079, -51.466) construction
  spline S169 degree 3 poles (-25.7079, -51.466) (-25.5697, -51.5975) (-25.5839, -51.7337) (-25.7338, -51.7142) knots 0 0 0 0 1 1 1 1
  line L526 (-25.7079, -51.466) -> (-25.5697, -51.5975) construction
  line L527 (-25.5697, -51.5975) -> (-25.5839, -51.7337) construction
  line L528 (-25.5839, -51.7337) -> (-25.7338, -51.7142) construction
  spline S170 degree 3 poles (-25.7338, -51.7142) (-26.021, -51.677) (-26.0573, -51.6823) (-26.1938, -51.7814) knots 0 0 0 0 1 1 1 1
  line L529 (-25.7338, -51.7142) -> (-26.021, -51.677) construction
  line L530 (-26.021, -51.677) -> (-26.0573, -51.6823) construction
  line L531 (-26.0573, -51.6823) -> (-26.1938, -51.7814) construction
  spline S171 degree 3 poles (-26.1938, -51.7814) (-26.2892, -51.8507) (-26.3698, -51.8748) (-26.4571, -51.8601) knots 0 0 0 0 1 1 1 1
  line L532 (-26.1938, -51.7814) -> (-26.2892, -51.8507) construction
  line L533 (-26.2892, -51.8507) -> (-26.3698, -51.8748) construction
  line L534 (-26.3698, -51.8748) -> (-26.4571, -51.8601) construction
  spline S172 degree 3 poles (-26.4571, -51.8601) (-26.5347, -51.847) (-26.636, -51.7649) (-26.636, -51.7152) knots 0 0 0 0 1 1 1 1
  line L535 (-26.4571, -51.8601) -> (-26.5347, -51.847) construction
  line L536 (-26.5347, -51.847) -> (-26.636, -51.7649) construction
  line L537 (-26.636, -51.7649) -> (-26.636, -51.7152) construction
  spline S173 degree 3 poles (-26.636, -51.7152) (-26.636, -51.67) (-26.4944, -51.5339) (-26.3468, -51.4371) knots 0 0 0 0 1 1 1 1
  line L538 (-26.636, -51.7152) -> (-26.636, -51.67) construction
  line L539 (-26.636, -51.67) -> (-26.4944, -51.5339) construction
  line L540 (-26.4944, -51.5339) -> (-26.3468, -51.4371) construction
  spline S174 degree 3 poles (-26.3468, -51.4371) (-26.1498, -51.3078) (-26.0886, -51.2992) (-25.8871, -51.3719) knots 0 0 0 0 1 1 1 1
  line L541 (-26.3468, -51.4371) -> (-26.1498, -51.3078) construction
  line L542 (-26.1498, -51.3078) -> (-26.0886, -51.2992) construction
  line L543 (-26.0886, -51.2992) -> (-25.8871, -51.3719) construction
  spline S175 degree 3 poles (-26.0634, -52.158) (-25.9586, -52.2673) (-25.9464, -52.3527) (-26.0324, -52.3743) knots 0 0 0 0 1 1 1 1
  line L544 (-26.0634, -52.158) -> (-25.9586, -52.2673) construction
  line L545 (-25.9586, -52.2673) -> (-25.9464, -52.3527) construction
  line L546 (-25.9464, -52.3527) -> (-26.0324, -52.3743) construction
  spline S176 degree 3 poles (-26.0324, -52.3743) (-26.0925, -52.3893) (-26.1704, -52.352) (-26.2006, -52.2936) knots 0 0 0 0 1 1 1 1
  line L547 (-26.0324, -52.3743) -> (-26.0925, -52.3893) construction
  line L548 (-26.0925, -52.3893) -> (-26.1704, -52.352) construction
  line L549 (-26.1704, -52.352) -> (-26.2006, -52.2936) construction
  spline S177 degree 3 poles (-26.2006, -52.2936) (-26.2394, -52.2186) (-26.2081, -52.0837) (-26.1519, -52.0837) knots 0 0 0 0 1 1 1 1
  line L550 (-26.2006, -52.2936) -> (-26.2394, -52.2186) construction
  line L551 (-26.2394, -52.2186) -> (-26.2081, -52.0837) construction
  line L552 (-26.2081, -52.0837) -> (-26.1519, -52.0837) construction
  spline S178 degree 3 poles (-26.1519, -52.0837) (-26.1424, -52.0837) (-26.1025, -52.1171) (-26.0634, -52.158) knots 0 0 0 0 1 1 1 1
  line L553 (-26.1519, -52.0837) -> (-26.1424, -52.0837) construction
  line L554 (-26.1424, -52.0837) -> (-26.1025, -52.1171) construction
  line L555 (-26.1025, -52.1171) -> (-26.0634, -52.158) construction
  spline S179 degree 3 poles (-26.2361, -38.0663) (-26.1877, -38.0906) (-25.9889, -38.2155) (-25.7816, -38.3237) knots 0 0 0 0 1 1 1 1
  line L556 (-26.2361, -38.0663) -> (-26.1877, -38.0906) construction
  line L557 (-26.1877, -38.0906) -> (-25.9889, -38.2155) construction
  line L558 (-25.9889, -38.2155) -> (-25.7816, -38.3237) construction
  spline S180 degree 3 poles (-25.7816, -38.3237) (-23.9688, -39.27) (-18.4738, -42.39) (-18.5268, -42.443) knots 0 0 0 0 1 1 1 1
  line L559 (-25.7816, -38.3237) -> (-23.9688, -39.27) construction
  line L560 (-23.9688, -39.27) -> (-18.4738, -42.39) construction
  line L561 (-18.4738, -42.39) -> (-18.5268, -42.443) construction
  spline S181 degree 3 poles (-18.5268, -42.443) (-18.5558, -42.4719) (-20.1846, -41.6459) (-22.2482, -40.5558) knots 0 0 0 0 1 1 1 1
  line L562 (-18.5268, -42.443) -> (-18.5558, -42.4719) construction
  line L563 (-18.5558, -42.4719) -> (-20.1846, -41.6459) construction
  line L564 (-20.1846, -41.6459) -> (-22.2482, -40.5558) construction
  spline S182 degree 3 poles (-22.2482, -40.5558) (-23.0823, -40.1151) (-24.6059, -39.2745) (-25.1085, -39.0397) knots 0 0 0 0 1 1 1 1
  line L565 (-22.2482, -40.5558) -> (-23.0823, -40.1151) construction
  line L566 (-23.0823, -40.1151) -> (-24.6059, -39.2745) construction
  line L567 (-24.6059, -39.2745) -> (-25.1085, -39.0397) construction
  spline S183 degree 3 poles (-25.1085, -39.0397) (-25.5432, -38.8365) (-25.9672, -38.5619) (-26.1123, -38.5179) knots 0 0 0 0 1 1 1 1
  line L568 (-25.1085, -39.0397) -> (-25.5432, -38.8365) construction
  line L569 (-25.5432, -38.8365) -> (-25.9672, -38.5619) construction
  line L570 (-25.9672, -38.5619) -> (-26.1123, -38.5179) construction
  spline S184 degree 3 poles (-26.1123, -38.5179) (-26.2586, -38.4734) (-26.285, -38.4448) (-26.6344, -38.6517) knots 0 0 0 0 1 1 1 1
  line L571 (-26.1123, -38.5179) -> (-26.2586, -38.4734) construction
  line L572 (-26.2586, -38.4734) -> (-26.285, -38.4448) construction
  line L573 (-26.285, -38.4448) -> (-26.6344, -38.6517) construction
  spline S185 degree 3 poles (-26.6344, -38.6517) (-27.3081, -39.0507) (-30.0851, -40.675) (-32.0319, -41.7706) knots 0 0 0 0 1 1 1 1
  line L574 (-26.6344, -38.6517) -> (-27.3081, -39.0507) construction
  line L575 (-27.3081, -39.0507) -> (-30.0851, -40.675) construction
  line L576 (-30.0851, -40.675) -> (-32.0319, -41.7706) construction
  spline S186 degree 3 poles (-32.0319, -41.7706) (-32.4955, -42.0314) (-33.0541, -42.3427) (-33.2732, -42.4624) knots 0 0 0 0 1 1 1 1
  line L577 (-32.0319, -41.7706) -> (-32.4955, -42.0314) construction
  line L578 (-32.4955, -42.0314) -> (-33.0541, -42.3427) construction
  line L579 (-33.0541, -42.3427) -> (-33.2732, -42.4624) construction
  spline S187 degree 3 poles (-33.2732, -42.4624) (-33.8333, -42.7682) (-33.8912, -42.7889) (-33.8912, -42.6831) knots 0 0 0 0 1 1 1 1
  line L580 (-33.2732, -42.4624) -> (-33.8333, -42.7682) construction
  line L581 (-33.8333, -42.7682) -> (-33.8912, -42.7889) construction
  line L582 (-33.8912, -42.7889) -> (-33.8912, -42.6831) construction
  spline S188 degree 3 poles (-33.8912, -42.6831) (-33.8912, -42.6467) (-33.8689, -42.6143) (-33.7962, -42.5451) knots 0 0 0 0 1 1 1 1
  line L583 (-33.8912, -42.6831) -> (-33.8912, -42.6467) construction
  line L584 (-33.8912, -42.6467) -> (-33.8689, -42.6143) construction
  line L585 (-33.8689, -42.6143) -> (-33.7962, -42.5451) construction
  spline S189 degree 3 poles (-33.7962, -42.5451) (-33.6077, -42.3657) (-33.2763, -42.1619) (-31.7179, -41.2671) knots 0 0 0 0 1 1 1 1
  line L586 (-33.7962, -42.5451) -> (-33.6077, -42.3657) construction
  line L587 (-33.6077, -42.3657) -> (-33.2763, -42.1619) construction
  line L588 (-33.2763, -42.1619) -> (-31.7179, -41.2671) construction
  spline S190 degree 3 poles (-31.7179, -41.2671) (-29.4107, -39.9422) (-27.7597, -38.9867) (-26.8602, -38.3838) knots 0 0 0 0 1 1 1 1
  line L589 (-31.7179, -41.2671) -> (-29.4107, -39.9422) construction
  line L590 (-29.4107, -39.9422) -> (-27.7597, -38.9867) construction
  line L591 (-27.7597, -38.9867) -> (-26.8602, -38.3838) construction
  spline S191 degree 3 poles (-26.8602, -38.3838) (-26.686, -38.2671) (-26.3952, -38.0674) (-26.3922, -38.0681) knots 0 0 0 0 1 1 1 1
  line L592 (-26.8602, -38.3838) -> (-26.686, -38.2671) construction
  line L593 (-26.686, -38.2671) -> (-26.3952, -38.0674) construction
  line L594 (-26.3952, -38.0674) -> (-26.3922, -38.0681) construction
  spline S192 degree 3 poles (-26.3922, -38.0681) (-26.3892, -38.0688) (-26.2936, -38.0375) (-26.2452, -38.0618) knots 0 0 0 0 1 1 1 1
  line L595 (-26.3922, -38.0681) -> (-26.3892, -38.0688) construction
  line L596 (-26.3892, -38.0688) -> (-26.2936, -38.0375) construction
  line L597 (-26.2936, -38.0375) -> (-26.2452, -38.0618) construction
  line L598 (-26.2452, -38.0618) -> (-26.2361, -38.0663)
  spline S193 degree 3 poles (-25.5701, -36.7497) (-24.7732, -37.2051) (-23.7509, -37.7809) (-21.4963, -39.0441) knots 0 0 0 0 1 1 1 1
  line L599 (-25.5701, -36.7497) -> (-24.7732, -37.2051) construction
  line L600 (-24.7732, -37.2051) -> (-23.7509, -37.7809) construction
  line L601 (-23.7509, -37.7809) -> (-21.4963, -39.0441) construction
  spline S194 degree 3 poles (-21.4963, -39.0441) (-20.4373, -39.6374) (-19.3961, -40.2233) (-19.1825, -40.3461) knots 0 0 0 0 1 1 1 1
  line L602 (-21.4963, -39.0441) -> (-20.4373, -39.6374) construction
  line L603 (-20.4373, -39.6374) -> (-19.3961, -40.2233) construction
  line L604 (-19.3961, -40.2233) -> (-19.1825, -40.3461) construction
  spline S195 degree 3 poles (-19.1825, -40.3461) (-18.2686, -40.8715) (-17.5092, -41.3427) (-17.5349, -41.3684) knots 0 0 0 0 1 1 1 1
  line L605 (-19.1825, -40.3461) -> (-18.2686, -40.8715) construction
  line L606 (-18.2686, -40.8715) -> (-17.5092, -41.3427) construction
  line L607 (-17.5092, -41.3427) -> (-17.5349, -41.3684) construction
  spline S196 degree 3 poles (-17.5349, -41.3684) (-17.5563, -41.3899) (-18.152, -41.1096) (-18.7942, -40.7758) knots 0 0 0 0 1 1 1 1
  line L608 (-17.5349, -41.3684) -> (-17.5563, -41.3899) construction
  line L609 (-17.5563, -41.3899) -> (-18.152, -41.1096) construction
  line L610 (-18.152, -41.1096) -> (-18.7942, -40.7758) construction
  spline S197 degree 3 poles (-18.7942, -40.7758) (-19.3152, -40.5051) (-19.5953, -40.3547) (-21.0433, -39.5686) knots 0 0 0 0 1 1 1 1
  line L611 (-18.7942, -40.7758) -> (-19.3152, -40.5051) construction
  line L612 (-19.3152, -40.5051) -> (-19.5953, -40.3547) construction
  line L613 (-19.5953, -40.3547) -> (-21.0433, -39.5686) construction
  spline S198 degree 3 poles (-21.0433, -39.5686) (-24.7068, -37.5796) (-25.5366, -37.1463) (-25.944, -37.0098) knots 0 0 0 0 1 1 1 1
  line L614 (-21.0433, -39.5686) -> (-24.7068, -37.5796) construction
  line L615 (-24.7068, -37.5796) -> (-25.5366, -37.1463) construction
  line L616 (-25.5366, -37.1463) -> (-25.944, -37.0098) construction
  spline S199 degree 3 poles (-25.944, -37.0098) (-26.1661, -36.9354) (-26.2273, -36.9431) (-26.3671, -37.0631) knots 0 0 0 0 1 1 1 1
  line L617 (-25.944, -37.0098) -> (-26.1661, -36.9354) construction
  line L618 (-26.1661, -36.9354) -> (-26.2273, -36.9431) construction
  line L619 (-26.2273, -36.9431) -> (-26.3671, -37.0631) construction
  spline S200 degree 3 poles (-26.3671, -37.0631) (-26.684, -37.3352) (-33.3641, -40.9778) (-34.4834, -41.4889) knots 0 0 0 0 1 1 1 1
  line L620 (-26.3671, -37.0631) -> (-26.684, -37.3352) construction
  line L621 (-26.684, -37.3352) -> (-33.3641, -40.9778) construction
  line L622 (-33.3641, -40.9778) -> (-34.4834, -41.4889) construction
  spline S201 degree 3 poles (-34.4834, -41.4889) (-34.656, -41.5677) (-34.6751, -41.573) (-34.7271, -41.5558) knots 0 0 0 0 1 1 1 1
  line L623 (-34.4834, -41.4889) -> (-34.656, -41.5677) construction
  line L624 (-34.656, -41.5677) -> (-34.6751, -41.573) construction
  line L625 (-34.6751, -41.573) -> (-34.7271, -41.5558) construction
  spline S202 degree 3 poles (-34.7271, -41.5558) (-34.7981, -41.5324) (-34.8332, -41.4831) (-34.8332, -41.4069) knots 0 0 0 0 1 1 1 1
  line L626 (-34.7271, -41.5558) -> (-34.7981, -41.5324) construction
  line L627 (-34.7981, -41.5324) -> (-34.8332, -41.4831) construction
  line L628 (-34.8332, -41.4831) -> (-34.8332, -41.4069) construction
  spline S203 degree 3 poles (-34.8332, -41.4069) (-34.8332, -41.3443) (-34.7852, -41.2753) (-34.7415, -41.2753) knots 0 0 0 0 1 1 1 1
  line L629 (-34.8332, -41.4069) -> (-34.8332, -41.3443) construction
  line L630 (-34.8332, -41.3443) -> (-34.7852, -41.2753) construction
  line L631 (-34.7852, -41.2753) -> (-34.7415, -41.2753) construction
  spline S204 degree 3 poles (-34.7415, -41.2753) (-34.6513, -41.2753) (-33.03, -40.3617) (-29.1481, -38.1236) knots 0 0 0 0 1 1 1 1
  line L632 (-34.7415, -41.2753) -> (-34.6513, -41.2753) construction
  line L633 (-34.6513, -41.2753) -> (-33.03, -40.3617) construction
  line L634 (-33.03, -40.3617) -> (-29.1481, -38.1236) construction
  spline S205 degree 3 poles (-29.1481, -38.1236) (-26.7717, -36.7534) (-26.1815, -36.4161) (-26.1631, -36.4178) knots 0 0 0 0 1 1 1 1
  line L635 (-29.1481, -38.1236) -> (-26.7717, -36.7534) construction
  line L636 (-26.7717, -36.7534) -> (-26.1815, -36.4161) construction
  line L637 (-26.1815, -36.4161) -> (-26.1631, -36.4178) construction
  spline S206 degree 3 poles (-26.1631, -36.4178) (-26.1551, -36.4185) (-25.8882, -36.5678) (-25.5701, -36.7497) knots 0 0 0 0 1 1 1 1
  line L638 (-26.1631, -36.4178) -> (-26.1551, -36.4185) construction
  line L639 (-26.1551, -36.4185) -> (-25.8882, -36.5678) construction
  line L640 (-25.8882, -36.5678) -> (-25.5701, -36.7497) construction
  spline S207 degree 3 poles (-25.6667, -35.9114) (-23.3942, -37.142) (-18.1096, -40.1031) (-17.426, -40.5288) knots 0 0 0 0 1 1 1 1
  line L641 (-25.6667, -35.9114) -> (-23.3942, -37.142) construction
  line L642 (-23.3942, -37.142) -> (-18.1096, -40.1031) construction
  line L643 (-18.1096, -40.1031) -> (-17.426, -40.5288) construction
  spline S208 degree 3 poles (-17.426, -40.5288) (-17.1962, -40.672) (-17.057, -40.7775) (-17.0962, -40.7788) knots 0 0 0 0 1 1 1 1
  line L644 (-17.426, -40.5288) -> (-17.1962, -40.672) construction
  line L645 (-17.1962, -40.672) -> (-17.057, -40.7775) construction
  line L646 (-17.057, -40.7775) -> (-17.0962, -40.7788) construction
  spline S209 degree 3 poles (-17.0962, -40.7788) (-17.193, -40.782) (-18.8165, -39.9439) (-21.0252, -38.7504) knots 0 0 0 0 1 1 1 1
  line L647 (-17.0962, -40.7788) -> (-17.193, -40.782) construction
  line L648 (-17.193, -40.782) -> (-18.8165, -39.9439) construction
  line L649 (-18.8165, -39.9439) -> (-21.0252, -38.7504) construction
  spline S210 degree 3 poles (-21.0252, -38.7504) (-24.5873, -36.8258) (-25.2904, -36.4572) (-25.7601, -36.2678) knots 0 0 0 0 1 1 1 1
  line L650 (-21.0252, -38.7504) -> (-24.5873, -36.8258) construction
  line L651 (-24.5873, -36.8258) -> (-25.2904, -36.4572) construction
  line L652 (-25.2904, -36.4572) -> (-25.7601, -36.2678) construction
  spline S211 degree 3 poles (-25.7601, -36.2678) (-25.9601, -36.1872) (-25.9961, -36.1778) (-26.1072, -36.1773) knots 0 0 0 0 1 1 1 1
  line L653 (-25.7601, -36.2678) -> (-25.9601, -36.1872) construction
  line L654 (-25.9601, -36.1872) -> (-25.9961, -36.1778) construction
  line L655 (-25.9961, -36.1778) -> (-26.1072, -36.1773) construction
  spline S212 degree 3 poles (-26.1072, -36.1773) (-26.2282, -36.1769) (-26.2336, -36.1786) (-26.3385, -36.2528) knots 0 0 0 0 1 1 1 1
  line L656 (-26.1072, -36.1773) -> (-26.2282, -36.1769) construction
  line L657 (-26.2282, -36.1769) -> (-26.2336, -36.1786) construction
  line L658 (-26.2336, -36.1786) -> (-26.3385, -36.2528) construction
  spline S213 degree 3 poles (-26.3385, -36.2528) (-26.5325, -36.3899) (-26.9027, -36.5968) (-28.0077, -37.1853) knots 0 0 0 0 1 1 1 1
  line L659 (-26.3385, -36.2528) -> (-26.5325, -36.3899) construction
  line L660 (-26.5325, -36.3899) -> (-26.9027, -36.5968) construction
  line L661 (-26.9027, -36.5968) -> (-28.0077, -37.1853) construction
  spline S214 degree 3 poles (-28.0077, -37.1853) (-29.0123, -37.7204) (-30.2741, -38.4093) (-31.8667, -39.2922) knots 0 0 0 0 1 1 1 1
  line L662 (-28.0077, -37.1853) -> (-29.0123, -37.7204) construction
  line L663 (-29.0123, -37.7204) -> (-30.2741, -38.4093) construction
  line L664 (-30.2741, -38.4093) -> (-31.8667, -39.2922) construction
  spline S215 degree 3 poles (-31.8667, -39.2922) (-34.6982, -40.862) (-35.1953, -41.1229) (-35.2871, -41.0877) knots 0 0 0 0 1 1 1 1
  line L665 (-31.8667, -39.2922) -> (-34.6982, -40.862) construction
  line L666 (-34.6982, -40.862) -> (-35.1953, -41.1229) construction
  line L667 (-35.1953, -41.1229) -> (-35.2871, -41.0877) construction
  spline S216 degree 3 poles (-35.2871, -41.0877) (-35.3031, -41.0816) (-35.3125, -41.057) (-35.3125, -41.021) knots 0 0 0 0 1 1 1 1
  line L668 (-35.2871, -41.0877) -> (-35.3031, -41.0816) construction
  line L669 (-35.3031, -41.0816) -> (-35.3125, -41.057) construction
  line L670 (-35.3125, -41.057) -> (-35.3125, -41.021) construction
  spline S217 degree 3 poles (-35.3125, -41.021) (-35.3125, -40.9561) (-35.289, -40.9344) (-35.0398, -40.768) knots 0 0 0 0 1 1 1 1
  line L671 (-35.3125, -41.021) -> (-35.3125, -40.9561) construction
  line L672 (-35.3125, -40.9561) -> (-35.289, -40.9344) construction
  line L673 (-35.289, -40.9344) -> (-35.0398, -40.768) construction
  spline S218 degree 3 poles (-35.0398, -40.768) (-34.1437, -40.1697) (-31.5928, -38.6629) (-29.8835, -37.7222) knots 0 0 0 0 1 1 1 1
  line L674 (-35.0398, -40.768) -> (-34.1437, -40.1697) construction